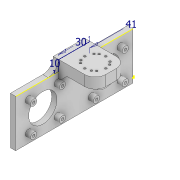
# Autodesk Inventor part: StereoVisionHolder_3
Saved by Autodesk Inventor 2022 (Build 260153000, 153)
## iProperties
Created: 2022-11-13
Part Number: StereoVisionHolder_3
Material: Generic
Document SubType Name: Modeling
Designer: MVeszpremi
Density: 1 g/cm^3
Appearance: Default
Author: MVeszpremi
Autodesk Inventor part; units mm, degrees
ref_plane "YZ Plane" through (0, 0, 0) normal (1, 0, 0) x (0, 1, 0)
ref_plane "XZ Plane" through (0, 0, 0) normal (0, 1, 0) x (-1, 0, 0)
ref_plane "XY Plane" through (0, 0, 0) normal (0, 0, 1) x (1, 0, 0)
sketch "Sketch1" plane through (0, 0, 0) normal (0, 0, 1) x (1, 0, 0)
  line L0 (0, 0) -> (20, 0)
  line L1 (20, 0) -> (20, 35)
  line L2 (20, 35) -> (0, 35)
  line L3 (0, 35) -> (0, 0)
  circle A0 centre (0, 35) radius 1.5
  circle A1 centre (20, 35) radius 1.5
  circle A2 centre (0, 0) radius 1.5
  circle A3 centre (20, 0) radius 1.5
  line L4 (0, 35) -> (20, 0)
  line L5 (-15, -5) -> (20, -5)
  line L6 (20, -5) -> (20, 40)
  line L7 (20, 40) -> (-15, 40)
  line L8 (-15, 40) -> (-15, -5)
  line L9 (20, 40) -> (25, 40)
  line L10 (25, 40) -> (25, -5)
  line L11 (25, -5) -> (20, -5)
  line L12 (20, -5) -> (20, 40)
  point P0 (10, 17.5)
  point P1 (20, 36.5)
  point P2 (20, 33.5)
  point P3 (20, 1.5)
  point P4 (20, -1.5)
  dimension "d0" = 35
  dimension "d1" = 20
  dimension "d2" = 3
  dimension "d3" = 3
  dimension "d4" = 3
  dimension "d5" = 3
  dimension "d6" = 5
  dimension "d7" = 15
  dimension "d45" = 5
  dimension "d46" = 45
  dimension "d47" = 10
  constraints: 26 end point, 6 parallel, 4 centre point, 4 coincident, 3 horizontal, 3 perpendicular, 1 midpoint
  measures "d0" distance of L2.end L0.start
  measures "d1" distance of L1.end L2.end
  measures "d2" diameter of A0
  measures "d3" diameter of A1
  measures "d4" diameter of A2
  measures "d5" diameter of A3
  measures "d6" distance between parallel lines of L2 L7
  measures "d7" distance between parallel lines of L8 L3
  measures "d45" distance of L6.end L9.end
  measures "d46" distance between parallel lines of L11 L9
  measures "d47" distance from line of L6 point (10, 17.5)
extrude "Extrusion1" add sketch "Sketch1" along normal blind 5 contours A2 L3 A0 L4 A3 L0 | L0 A3 L6 L5 L8 L7 A1 L2 A0 L3 A2 | L4 A0 L2 A1 L1 A3 | A3 L1 A1 L6 L9 L10 L11
sketch "Sketch2" plane through (0, 0, 5) normal (0, 0, 1) x (1, 0, 0)
  line L0 (30, 40) -> (-15, 40) projected
  line L1 (-15, 40) -> (-20, 40)
  line L2 (-20, 40) -> (-20, -5)
  line L3 (-20, -5) -> (-15, -5)
  line L4 (-15, -5) -> (-15, 40)
  point P0 (0, 0)
  dimension "d10" = 5
  constraints: 8 end point, 2 parallel, 1 coincident, 1 horizontal, 1 perpendicular
  measures "d10" distance of L0.end L1.end
extrude "Extrusion2" add sketch "Sketch2" along normal blind 107 and the other way blind 5
ref_plane "Work Plane2" through (0, 0, 56) normal (0, 0, -1) x (-1, 0, 0)
mirror "Mirror2" about plane through (0, 0, 56) normal (0, 0, -1) of "Extrusion1"
sketch "Sketch3" plane through (-15, -5, 5) normal (1, 0, 0) x (0, 0, -1)
  line L0 (-102, 45) -> (-102, 0) projected
  line L1 (-102, 22.5) -> (0, 22.5)
  line L2 (0, 45) -> (0, 0) projected
  circle A0 centre (-81, 22.5) radius 13.5
  circle A1 centre (-21, 22.5) radius 13.5
  line L3 (-94.75, 36.25) -> (-67.25, 36.25)
  line L4 (-67.25, 36.25) -> (-67.25, 8.75)
  line L5 (-67.25, 8.75) -> (-94.75, 8.75)
  line L6 (-94.75, 8.75) -> (-94.75, 36.25)
  line L7 (-94.75, 36.25) -> (-67.25, 8.75) construction
  line L8 (-67.25, 36.25) -> (-94.75, 8.75) construction
  line L9 (0, 45) -> (-102, 45) projected
  line L10 (-7.25, 8.75) -> (-34.75, 8.75)
  line L11 (-34.75, 8.75) -> (-34.75, 36.25)
  line L12 (-34.75, 36.25) -> (-7.25, 36.25)
  line L13 (-7.25, 36.25) -> (-7.25, 8.75)
  line L14 (-7.25, 8.75) -> (-34.75, 36.25) construction
  line L15 (-34.75, 8.75) -> (-7.25, 36.25) construction
  circle A2 centre (-94.75, 36.25) radius 3
  circle A3 centre (-67.25, 36.25) radius 3
  circle A4 centre (-67.25, 8.75) radius 3
  circle A5 centre (-94.75, 8.75) radius 3
  circle A6 centre (-34.75, 36.25) radius 3
  circle A7 centre (-7.25, 36.25) radius 3
  circle A8 centre (-7.25, 8.75) radius 3
  circle A9 centre (-34.75, 8.75) radius 3
  circle A10 centre (-94.75, 36.25) radius 1.25
  circle A11 centre (-67.25, 36.25) radius 1.25
  circle A12 centre (-67.25, 8.75) radius 1.25
  circle A13 centre (-94.75, 8.75) radius 1.25
  circle A14 centre (-34.75, 36.25) radius 1.25
  circle A15 centre (-7.25, 36.25) radius 1.25
  circle A16 centre (-34.75, 8.75) radius 1.25
  circle A17 centre (-7.25, 8.75) radius 1.25
  point P0 (5, 5)
  dimension "d16" = 27
  dimension "d17" = 27
  dimension "d18" = 27.5
  dimension "d19" = 27.5
  dimension "d20" = 22.5
  dimension "d21" = 21
  dimension "d22" = 21
  dimension "d23" = 27.5
  dimension "d24" = 27.5
  dimension "d25" = 6
  dimension "d26" = 6
  dimension "d27" = 6
  dimension "d28" = 6
  dimension "d29" = 6
  dimension "d30" = 6
  dimension "d31" = 6
  dimension "d32" = 6
  dimension "d33" = 2.5
  dimension "d34" = 2.5
  dimension "d35" = 2.5
  dimension "d36" = 2.5
  dimension "d37" = 2.5
  dimension "d38" = 2.5
  dimension "d39" = 2.5
  dimension "d40" = 2.5
  constraints: 26 end point, 18 centre point, 16 coincident, 6 midpoint, 4 parallel, 3 horizontal, 2 perpendicular, 2 point on line
  measures "d16" diameter of A0
  measures "d17" diameter of A1
  measures "d18" distance of L4.end L5.end
  measures "d19" distance of L3.end L4.end
  measures "d20" distance between parallel lines of L9 L1
  measures "d21" distance from line of L0 A0.centre
  measures "d22" distance from line of L2 A1.centre
  measures "d23" distance of L11.end L12.end
  measures "d24" distance of L10.end L11.end
  measures "d25" diameter of A3
  measures "d26" diameter of A2
  measures "d27" diameter of A5
  measures "d28" diameter of A4
  measures "d29" diameter of A9
  measures "d30" diameter of A6
  measures "d31" diameter of A7
  measures "d32" diameter of A8
  measures "d33" diameter of A10
  measures "d34" diameter of A11
  measures "d35" diameter of A12
  measures "d36" diameter of A13
  measures "d37" diameter of A14
  measures "d38" diameter of A15
  measures "d39" diameter of A16
  measures "d40" diameter of A17
extrude "Extrusion3" cut sketch "Sketch3" against normal blind 6 contours A0 L1 | L1 A0 | A13 L5 L6 | L6 L5 A13 | A10 L3 L6 | L6 L3 A10 | A1 L1 | L1 A1 | A15 L12 L13 | L13 L12 A15 | A17 L10 L13 | L13 L10 A17 | A12 L4 L5 | L5 L4 A12 | A11 L4 L3 | L3 L4 A11 | A14 L11 L12 | L12 L11 A14 | A16 L11 L10 | L10 L11 A16
extrude "Extrusion4" add sketch "Sketch3" along normal blind 5 contours A5 L5 A13 L6 | L6 A13 L5 A5 | A2 L3 A10 L6 | L6 A10 L3 A2 | A7 L12 A15 L13 | L13 A15 L12 A7 | A8 L10 A17 L13 | L13 A17 L10 A8 | A4 L4 A12 L5 | L5 A12 L4 A4 | A3 L4 A11 L3 | L3 A11 L4 A3 | A6 L11 A14 L12 | L12 A14 L11 A6 | A9 L11 A16 L10 | L10 A16 L11 A9
sketch "Sketch4" plane through (25, -5, 0) normal (1, 0, 0) x (0, 0, -1)
  line L0 (-112, 0) -> (-112, 45) projected
  line L1 (-112, 0) -> (-107, 0) projected
  line L2 (-107, 0) -> (-107, 45) projected
  line L3 (-112, 45) -> (-107, 45) projected
  line L4 (0, 0) -> (0, 45) projected
  line L5 (0, 45) -> (-5, 45) projected
  line L6 (-5, 0) -> (-5, 45) projected
  line L7 (0, 0) -> (-5, 0) projected
  point P0 (0, 5)
extrude "Extrusion5" cut sketch "Sketch4" against normal up to surface (40 mm away)
sketch "Sketch5" plane through (-15, -5, 0) normal (1, 0, 0) x (0, 0, -1)
  line L0 (-112, 45) -> (0, 45) projected
  line L1 (-71, 45) -> (-41, 45)
  line L2 (-41, 45) -> (-41, 55)
  line L3 (-41, 55) -> (-71, 55)
  line L4 (-71, 55) -> (-71, 45)
  point P0 (0, 5)
  point P1 (-41, 45)
  dimension "d51" = 30
  dimension "d52" = 41
  dimension "d53" = 10
  constraints: 8 end point, 2 parallel, 1 horizontal, 1 perpendicular, 1 point on line
  measures "d51" distance of L2.end L3.end
  measures "d52" distance of L0.end L1.end
  measures "d53" distance of L3.end L1.start
extrude "Extrusion6" add sketch "Sketch5" against normal up to surface (5 mm away)
extrude "Extrusion7" add sketch "Sketch5" along normal blind 35
sketch "Sketch6" plane through (-15, 40, 41) normal (0, -1, 0) x (1, 0, 0)
  line L0 (35, 30) -> (35, 0) projected
  line L1 (35, 15) -> (20, 15)
  circle A0 centre (20, 15) radius 10
  circle A1 centre (30, 15) radius 1
  circle A2 centre (20, 25) radius 1
  circle A3 centre (10, 15) radius 1
  circle A4 centre (20, 5) radius 1
  circle A5 centre (28.6603, 10) radius 1
  line L2 (20, 15) -> (28.6603, 10)
  line L3 (20, 15) -> (26.4279, 7.3396)
  circle A6 centre (26.4279, 7.3396) radius 1
  circle A7 centre (25, 23.6603) radius 1
  circle A8 centre (27.6604, 21.4279) radius 1
  circle A9 centre (11.3397, 20) radius 1
  circle A10 centre (13.5721, 22.6604) radius 1
  circle A11 centre (15, 6.3397) radius 1
  circle A12 centre (12.3396, 8.5721) radius 1
  point P0 (15, -41)
  dimension "d58" = 20
  dimension "d59" = 15
  dimension "d60" = 2
  dimension "d63" = 360
  dimension "d65" = 30
  dimension "d66" = 2
  dimension "d67" = 2
  dimension "d68" = 50
  dimension "d71" = 360
  constraints: 13 centre point, 6 end point, 3 point on circle, 2 coincident, 1 horizontal, 1 midpoint, 1 point on line, 26 other
  measures "d58" diameter of A0
  measures "d59" distance of L1.start L1.end
  measures "d60" diameter of A1
  measures "d65" angle of L1 L2
  measures "d66" diameter of A5
  measures "d67" diameter of A6
  measures "d68" angle of L1 L3
extrude "Extrusion8" cut sketch "Sketch6" against normal blind 35 contours A1 A0 L1 | L1 A0 A1 | A0 A1 L1 | L1 A1 A0 | A8 A0 | A0 A8 | A5 A0 | A0 L2 A5 | A0 A5 L2 | A6 A0 L3 | L3 A0 A6 | A7 A0 | A0 A7 | A0 A6 | A4 A0 | A0 A4 | A2 A0 | A0 A2 | A11 A0 | A0 A11 | A10 A0 | A0 A10 | A12 A0 | A0 A12 | A9 A0 | A0 A9 | A3 A0 | A0 A3
fillet "Fillet3" radius 10 2 edges at (20, 45, 71) (20, 45, 41)
chamfer "Chamfer1" distance 8 angle 45 1 edges at (-15, 40, 56)
fillet "Fillet4" radius 10 2 edges at (-17.5, 40, 71) (-17.5, 40, 41)
equation "\"d41\" = d30"
body "Solid1"
